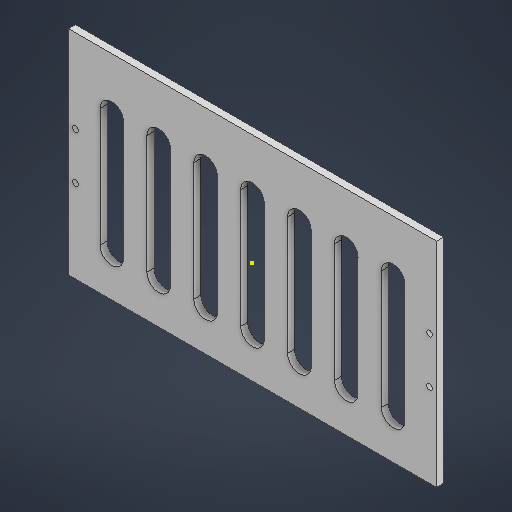
# Autodesk Inventor part: 后板3
Saved by Autodesk Inventor 2025 (Build 290162000, 162)
## iProperties
Created: 2024-12-27
Part Number: 后板3
Material: 常规
Document SubType Name: Modeling
Designer: HZD
Density: 1 g/cm^3
Appearance: 默认
Author: HZD
Autodesk Inventor part; units mm, degrees
ref_plane "YZ Plane" through (0, 0, 0) normal (1, 0, 0) x (0, 1, 0)
ref_plane "XZ Plane" through (0, 0, 0) normal (0, 1, 0) x (-1, 0, 0)
ref_plane "XY Plane" through (0, 0, 0) normal (0, 0, 1) x (1, 0, 0)
sketch "草图1" plane through (0, 0, 0) normal (0, 0, 1) x (1, 0, 0)
  line L0 (78.5, -47.5) -> (-78.5, -47.5)
  line L1 (-78.5, -47.5) -> (-78.5, 47.5)
  line L2 (-78.5, 47.5) -> (78.5, 47.5)
  line L3 (78.5, 47.5) -> (78.5, -47.5)
  line L4 (78.5, -47.5) -> (-78.5, 47.5) construction
  line L5 (-78.5, -47.5) -> (78.5, 47.5) construction
  point P0 (0, 0)
  dimension "d1" = 157
  dimension "d5" = 95
  constraints: 12 end point, 2 midpoint, 2 parallel, 1 horizontal, 1 perpendicular
  measures "d1" distance of L1.end L2.end
  measures "d5" distance of L0.end L1.end
extrude "拉伸1" add sketch "草图1" along normal blind 3
sketch "草图2" plane through (0, 0, 3) normal (0, 0, 1) x (1, 0, 0)
  point P0 (0, 0)
sketch "草图3" plane through (0, 0, 3) normal (0, 0, 1) x (1, 0, 0)
  line L0 (-79.9462, -43.4706) -> (81.0538, -43.4706)
  line L1 (78.5, 47.5) -> (-78.5, 47.5) projected
  line L2 (-78.5, 47.5) -> (-78.5, -47.5) projected
  line L3 (-78.5, -47.5) -> (78.5, -47.5) projected
  line L4 (78.5, -47.5) -> (78.5, 47.5) projected
  point P0 (0, 0)
  point P1 (78.5, -43.4706)
  point P2 (-78.5, -43.4706)
  constraints: 2 end point
extrude "拉伸2" cut sketch "草图3" against normal blind 10 contours L0 L4 L3 L2
sketch "草图4" plane through (0, 0, 0) normal (0, 0, -1) x (-1, 0, 0)
  circle A0 centre (-75.5, 11.9042) radius 1.2 projected
  ellipse E0 centre (-75.5, -7.8467) end of major axis (-76.7, -7.8467) minor radius 1.1265 projected
  circle A1 centre (75.5, 11.9042) radius 1.2 projected
  circle A2 centre (75.5, -8.0958) radius 1.2 projected
  point P0 (0, 0)
  constraints: 1 other
extrude "拉伸3" cut sketch "草图4" against normal blind 10
sketch "草图5" plane through (0, 0, 3) normal (0, 0, 1) x (1, 0, 0)
  line L0 (-60, 24.7542) -> (-60, -25.6955) construction
  line L1 (-65, 24.7542) -> (-65, -25.6955)
  line L2 (-55, -25.6955) -> (-55, 24.7542)
  arc A0 (-55, 24.7542) -> (-65, 24.7542) centre (-60, 24.7542) ccw
  arc A1 (-65, -25.6955) -> (-55, -25.6955) centre (-60, -25.6955) ccw
  line L3 (-78.5, -43.4706) -> (78.5, -43.4706) projected
  line L4 (-40, 24.7542) -> (-40, -25.6955) construction
  line L5 (-45, 24.7542) -> (-45, -25.6955)
  line L6 (-35, -25.6955) -> (-35, 24.7542)
  arc A2 (-35, 24.7542) -> (-45, 24.7542) centre (-40, 24.7542) ccw
  arc A3 (-45, -25.6955) -> (-35, -25.6955) centre (-40, -25.6955) ccw
  line L7 (-20, 24.7542) -> (-20, -25.6955) construction
  line L8 (-25, 24.7542) -> (-25, -25.6955)
  line L9 (-15, -25.6955) -> (-15, 24.7542)
  arc A4 (-15, 24.7542) -> (-25, 24.7542) centre (-20, 24.7542) ccw
  arc A5 (-25, -25.6955) -> (-15, -25.6955) centre (-20, -25.6955) ccw
  line L10 (0, 24.7542) -> (0, -25.6955) construction
  line L11 (-5, 24.7542) -> (-5, -25.6955)
  line L12 (5, -25.6955) -> (5, 24.7542)
  arc A6 (5, 24.7542) -> (-5, 24.7542) centre (0, 24.7542) ccw
  arc A7 (-5, -25.6955) -> (5, -25.6955) centre (0, -25.6955) ccw
  line L13 (20, 24.7542) -> (20, -25.6955) construction
  line L14 (15, 24.7542) -> (15, -25.6955)
  line L15 (25, -25.6955) -> (25, 24.7542)
  arc A8 (25, 24.7542) -> (15, 24.7542) centre (20, 24.7542) ccw
  arc A9 (15, -25.6955) -> (25, -25.6955) centre (20, -25.6955) ccw
  line L16 (40, 24.7542) -> (40, -25.6955) construction
  line L17 (35, 24.7542) -> (35, -25.6955)
  line L18 (45, -25.6955) -> (45, 24.7542)
  arc A10 (45, 24.7542) -> (35, 24.7542) centre (40, 24.7542) ccw
  arc A11 (35, -25.6955) -> (45, -25.6955) centre (40, -25.6955) ccw
  line L19 (60, 24.7542) -> (60, -25.6955) construction
  line L20 (55, 24.7542) -> (55, -25.6955)
  line L21 (65, -25.6955) -> (65, 24.7542)
  arc A12 (65, 24.7542) -> (55, 24.7542) centre (60, 24.7542) ccw
  arc A13 (55, -25.6955) -> (65, -25.6955) centre (60, -25.6955) ccw
  line L22 (80, 24.7542) -> (80, -25.6955) construction
  line L23 (75, 24.7542) -> (75, -25.6955)
  line L24 (85, -25.6955) -> (85, 24.7542)
  arc A14 (85, 24.7542) -> (75, 24.7542) centre (80, 24.7542) ccw
  arc A15 (75, -25.6955) -> (85, -25.6955) centre (80, -25.6955) ccw
  line L25 (100, 24.7542) -> (100, -25.6955) construction
  line L26 (95, 24.7542) -> (95, -25.6955)
  line L27 (105, -25.6955) -> (105, 24.7542)
  arc A16 (105, 24.7542) -> (95, 24.7542) centre (100, 24.7542) ccw
  arc A17 (95, -25.6955) -> (105, -25.6955) centre (100, -25.6955) ccw
  line L28 (120, 24.7542) -> (120, -25.6955) construction
  line L29 (115, 24.7542) -> (115, -25.6955)
  line L30 (125, -25.6955) -> (125, 24.7542)
  arc A18 (125, 24.7542) -> (115, 24.7542) centre (120, 24.7542) ccw
  arc A19 (115, -25.6955) -> (125, -25.6955) centre (120, -25.6955) ccw
  line L31 (-78.5, 47.5) -> (-78.5, -43.4706) projected
  line L32 (78.5, -43.4706) -> (78.5, 47.5) projected
  point P0 (0, 0)
  point P1 (-60, -0.4706)
  point P2 (-40, -0.4706)
  point P3 (-20, -0.4706)
  point P4 (0, -0.4706)
  point P5 (20, -0.4706)
  point P6 (40, -0.4706)
  point P7 (60, -0.4706)
  point P8 (80, -0.4706)
  point P9 (100, -0.4706)
  point P10 (120, -0.4706)
  dimension "d10" = 10
  dimension "d11" = 43
  dimension "d17" = 20
  dimension "d21" = 13.5
  dimension "d22" = 13.5
  constraints: 80 end point, 40 point on circle, 20 centre point, 4 tangent, 1 horizontal, 1 midpoint, 1 parallel, 1 vertical, 108 other
  measures "d10" distance between parallel lines of L2 L1
  measures "d11" distance from line of point (-60, -0.471) L3
  measures "d17" distance of L1.start L5.start
  measures "d21" distance between parallel lines of L1 L31
  measures "d22" distance between parallel lines of L32 L21
extrude "拉伸4" cut sketch "草图5" against normal blind 73.5 contours A0 L2 A1 L1 | A2 L6 A3 L5 | A4 L9 A5 L8 | A6 L12 A7 L11 | A8 L15 A9 L14 | A10 L18 A11 L17 | A12 L21 A13 L20
